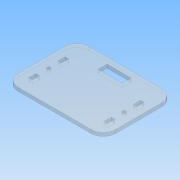
# Autodesk Inventor part: Front_panel
Saved by Autodesk Inventor 2016 (Build 200138000, 138)
## iProperties
Created: 2016-04-03
Part Number: Front_panel
Material: Polycarbonate, Clear
Document SubType Name: Modeling
Designer: admin
Density: 1.2 g/cm^3
Appearance: Polycarbonate - Clear
Author: admin
Autodesk Inventor part; units mm, degrees
ref_plane "YZ Plane" through (0, 0, 0) normal (1, 0, 0) x (0, 1, 0)
ref_plane "XZ Plane" through (0, 0, 0) normal (0, 1, 0) x (-1, 0, 0)
ref_plane "XY Plane" through (0, 0, 0) normal (0, 0, 1) x (1, 0, 0)
sketch "Sketch1" plane through (0, 0, 0) normal (0, 0, 1) x (1, 0, 0)
  line L0 (-30, 29) -> (30, 29)
  line L1 (40, 19) -> (40, -19)
  line L2 (30, -29) -> (-30, -29)
  line L3 (-40, -19) -> (-40, 19)
  arc A0 (-30, 29) -> (-40, 19) centre (-30, 19) ccw
  arc A1 (40, 19) -> (30, 29) centre (30, 19) ccw
  arc A2 (-40, -19) -> (-30, -29) centre (-30, -19) ccw
  arc A3 (30, -29) -> (40, -19) centre (30, -19) ccw
  line L4 (-10, 24) -> (10, 24)
  line L5 (10, 24) -> (10, 16.5)
  line L6 (10, 16.5) -> (-10, 16.5)
  line L7 (-10, 16.5) -> (-10, 24)
  point P0 (0, 0)
  point P1 (-40, 29)
  point P2 (40, -29)
  point P3 (40, 29)
  point P4 (-40, -29)
  point P5 (40, 0)
  point P6 (0, 29)
  point P7 (0, 16.5)
  dimension "d0" = 58
  dimension "d1" = 80
  dimension "d4" = 10
  dimension "d13" = 5
  dimension "d14" = 7.5
  dimension "d15" = 20
  constraints: 16 end point, 8 point on circle, 8 point on line, 8 tangent, 4 centre point, 4 parallel, 3 equal radius, 3 midpoint, 2 horizontal, 2 perpendicular, 2 vertical alignment, 1 horizontal alignment
  measures "d0" distance of point (40, 29) point (40, -29)
  measures "d1" distance of point (40, -29) point (-40, -29)
  measures "d4" radius of A0
  measures "d13" distance between parallel lines of L0 L4
  measures "d14" distance of L6.end L4.start
  measures "d15" distance of L5.end L6.end
extrude "Extrusion1" add sketch "Sketch1" along normal blind 3
sketch "Sketch2" plane through (0, 0, 3) normal (0, 0, 1) x (1, 0, 0)
  line L0 (30, 29) -> (-30, 29) projected
  arc A0 (-30, 29) -> (-40, 19) centre (-30, 19) ccw projected
  line L1 (-40, 19) -> (-40, -19) projected
  arc A1 (-40, -19) -> (-30, -29) centre (-30, -19) ccw projected
  line L2 (-30, -29) -> (30, -29) projected
  arc A2 (30, -29) -> (40, -19) centre (30, -19) ccw projected
  line L3 (40, -19) -> (40, 19) projected
  arc A3 (40, 19) -> (30, 29) centre (30, 19) ccw projected
  line L4 (-32.5, -18) -> (-29.5, -18)
  line L5 (-29.5, -18) -> (-29.5, -12)
  line L6 (-29.5, -12) -> (-32.5, -12)
  line L7 (-32.5, -12) -> (-32.5, -18)
  line L8 (-32.5, 6) -> (-29.5, 6)
  line L9 (-29.5, 6) -> (-29.5, 12)
  line L10 (-29.5, 12) -> (-32.5, 12)
  line L11 (-32.5, 12) -> (-32.5, 6)
  line L12 (29.5, -18) -> (32.5, -18)
  line L13 (32.5, -18) -> (32.5, -12)
  line L14 (32.5, -12) -> (29.5, -12)
  line L15 (29.5, -12) -> (29.5, -18)
  line L16 (29.5, 6) -> (32.5, 6)
  line L17 (32.5, 6) -> (32.5, 12)
  line L18 (32.5, 12) -> (29.5, 12)
  line L19 (29.5, 12) -> (29.5, 6)
  line L20 (-31, 6) -> (-31, -12) construction
  point P0 (0, 0)
  point P1 (-31, -3)
  point P2 (31, -3)
  point P3 (31, 6)
  point P4 (-31, -3)
  dimension "d5" = 62
  dimension "d17" = 31
  dimension "d18" = 3
  dimension "d19" = 6
  dimension "d20" = 3
  dimension "d21" = 18
  constraints: 34 end point, 8 parallel, 4 equal length, 4 horizontal, 4 midpoint, 4 perpendicular, 4 point on line, 2 collinear, 2 vertical alignment, 1 coincident, 1 horizontal alignment
  measures "d5" distance of point (31, -3) point (-31, -3)
  measures "d17" horizontal distance of point (0, 0) point (31, -3)
  measures "d18" vertical distance of point (-31, -3) point (0, 0)
  measures "d19" distance of L8.end L9.end
  measures "d20" distance of L9.end L10.end
  measures "d21" distance between parallel lines of L6 L8
hole "Hole1" at (-31, -3, 3) at (31, -3, 3) direction (0, 0, -1) diameter 3 end through all
extrude "Extrusion2" cut sketch "Sketch2" against normal up to next contours L7 L6 L5 L4 | L11 L10 L9 L8 | L15 L14 L13 L12 | L19 L18 L17 L16
equation "\"d17\" = 0.5 * d5"
body "Solid1"
